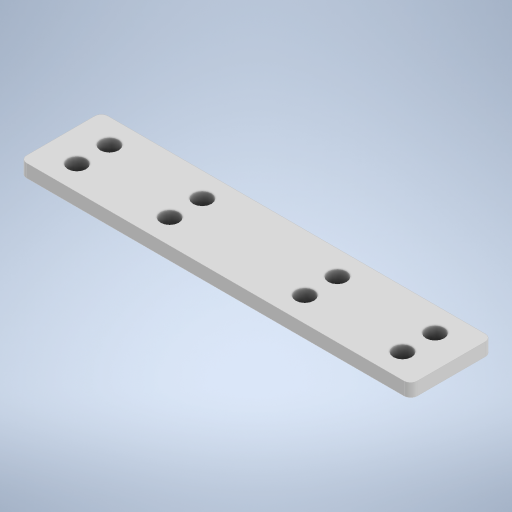
# Autodesk Inventor part: belka_wzdluz
Saved by Autodesk Inventor 2024.2 (Build 282272000, 272)
## iProperties
Created: 2024-01-11
Part Number: belka_wzdluz
Material: PLA
Document SubType Name: Modeling
Designer: Konrad
Density: 1 g/cm^3
Appearance: PLA
Author: Konrad
Autodesk Inventor part; units mm, degrees
ref_plane "YZ Plane" through (0, 0, 0) normal (1, 0, 0) x (0, 1, 0)
ref_plane "XZ Plane" through (0, 0, 0) normal (0, 1, 0) x (-1, 0, 0)
ref_plane "XY Plane" through (0, 0, 0) normal (0, 0, 1) x (1, 0, 0)
sketch "Szkic1" plane through (0, 0, 0) normal (0, 1, 0) x (-1, 0, 0)
  line L0 (0, 0) -> (80, 0)
  line L1 (80, 0) -> (80, -25)
  line L2 (80, -25) -> (0, -25)
  line L3 (0, -25) -> (0, 0)
  line L4 (80, -12.5) -> (0, -12.5) construction
  circle A0 centre (61.5, -7.5) radius 2.8
  circle A1 centre (61.5, -17.5) radius 2.8
  circle A2 centre (20, -7.5) radius 2.8
  circle A3 centre (20, -17.5) radius 2.8
  line L5 (80, 0) -> (100, 0)
  line L6 (100, 0) -> (100, -25)
  line L7 (100, -25) -> (80, -25)
  line L8 (80, -25) -> (80, 0)
  line L9 (0, 0) -> (-20, 0)
  line L10 (-20, 0) -> (-20, -25)
  line L11 (-20, -25) -> (0, -25)
  line L12 (0, -25) -> (0, 0)
  circle A4 centre (-10, -7.5) radius 2.8
  circle A5 centre (-10, -17.5) radius 2.8
  circle A6 centre (90, -7.5) radius 2.8
  circle A7 centre (90, -17.5) radius 2.8
  dimension "d0" = 80
  dimension "d1" = 25
  dimension "d2" = 5.6
  dimension "d3" = 10
  dimension "d4" = 20
  dimension "d5" = 18.5
  dimension "d6" = 10
  dimension "d9" = 20
  dimension "d10" = 20
  dimension "d12" = 10
  dimension "d13" = 10
  dimension "d14" = 10
  dimension "d15" = 10
  constraints: 26 end point, 8 centre point, 7 equal radius, 6 parallel, 4 symmetric about line, 3 horizontal, 3 perpendicular, 2 midpoint
  measures "d0" distance of L1.end L2.end
  measures "d1" distance of L0.end L1.end
  measures "d2" diameter of A0
  measures "d3" distance of A1.centre A0.centre
  measures "d4" distance from line of L3 A2.centre
  measures "d5" distance from line of L1 A0.centre
  measures "d6" distance of A3.centre A2.centre
  measures "d9" distance of L1.end L6.end
  measures "d10" distance of L2.end L10.end
  measures "d12" distance of A7.centre A6.centre
  measures "d13" distance of A5.centre A4.centre
  measures "d14" distance from line of L10 A5.centre
  measures "d15" distance from line of L1 A7.centre
extrude "Wyciągnięcie proste1" add sketch "Szkic1" along normal blind 4
fillet "Zaokrąglenie1" radius 2 4 edges at (-100, 2, 0) (20, 2, 0) (20, 2, -25) (-100, 2, -25)
equation "\"d6\" = d3"
equation "\"d13\" = d3"
equation "\"d14\" = 0.5 * d10"
equation "\"d15\" = 0.5 * d9"
